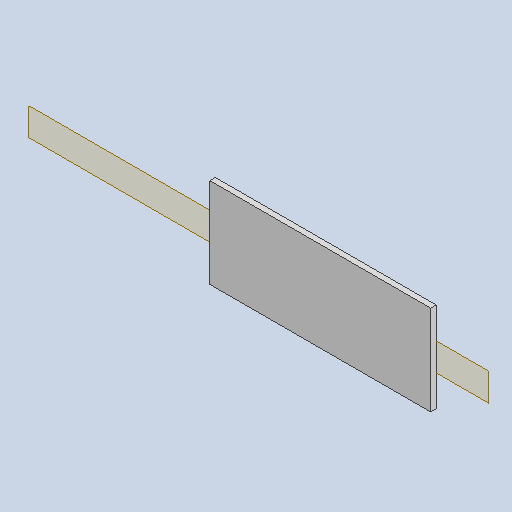
# Autodesk Inventor part: LAMINA_PARA_OREJA_DE_IZAJE
Saved by Autodesk Inventor 2023 (Build 270158000, 158)
## iProperties
RuleStatus: InUse
Created: 2023-06-02
Part Number: LAMINA_PARA_OREJA_DE_IZAJE
Material: Genérico
Document SubType Name: Sheet Metal
Designer: NELSON ORTIZ
Density: 1 g/cm^3
Sheet Metal Rule: Por defecto
Appearance: Valor por defecto
AfterDocOpen0: Regla0
AfterAnyParamChange0: Regla0
AfterAnyUserParamChange0: Regla0
Author: NELSON ORTIZ
Autodesk Inventor part; units mm, degrees
ref_plane "YZ Plane" through (0, 0, 0) normal (1, 0, 0) x (0, 1, 0)
ref_plane "XZ Plane" through (0, 0, 0) normal (0, 1, 0) x (-1, 0, 0)
ref_plane "XY Plane" through (0, 0, 0) normal (0, 0, 1) x (1, 0, 0)
ref_plane "Plano de trabajo1" through (316.0132, -51.5896, -104.0101) normal (0, 0, 1) x (1, 0, 0)
sketch "Boceto1" plane through (316.0132, -51.5896, -104.0101) normal (0, 0, 1) x (1, 0, 0)
  line L0 (-90, 23) -> (-270, 23) construction
  line L1 (-270, 9) -> (-270, 23) construction
  line L2 (-90, 9) -> (-270, 9) construction
  line L3 (-90, 9) -> (-90, 23) construction
  line L4 (-320, 73) -> (-40, 73)
  line L5 (-40, 73) -> (-40, -41)
  line L6 (-40, -41) -> (-320, -41)
  line L7 (-320, -41) -> (-320, 73)
  point P0 (-316.0132, 51.5896)
  dimension "d0" = 50
  measures "d0" distance between parallel lines of L0 L4
extrude "Placa1" add sketch "Boceto1" along normal blind 7
equation "\"d1\" = Grosor"
equation "\"Grosor\" = eb"
equation "\"Radio_pliegue\" = Grosor"
equation "\"Anchura_desahogo_plegado\" = Grosor"
equation "\"Profundidad_desahogo_plegado\" = 0.5 * Grosor"
equation "\"Tamaño_destalonado\" = 4 * Grosor"
equation "\"Remanente_mínimo\" = 2 * Grosor"
equation "\"Radiodetransición\" = Radio_pliegue"
equation "\"Tamaño_de_radio_de_Jacobi\" = Radio_pliegue"
equation "\"TamañoSeparación\" = Grosor"
equation "\"eb\" = 7"
